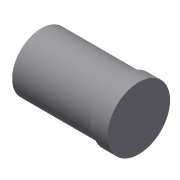
# Autodesk Inventor part: 00_Berrybase_CCTVLens_100mm
Saved by Autodesk Inventor 2022 (Build 260153000, 153)
## iProperties
Created: 2022-08-01
Part Number: 00_Berrybase_CCTVLens_100mm
Material: Generisch
Document SubType Name: Modeling
Designer: diederichbenedict
Density: 1 g/cm^3
Appearance: Vorgabe
Author: diederichbenedict
Autodesk Inventor part; units mm, degrees
ref_plane "YZ Plane" through (0, 0, 0) normal (1, 0, 0) x (0, 1, 0)
sketch "Skizze1" plane through (0, 0, 0) normal (0, 1, 0) x (-1, 0, 0)
  line L0 (0, 0) -> (0, -21)
  line L1 (0, -21) -> (9.5, -21)
  line L2 (9.5, -21) -> (13.5, -19.5)
  line L3 (13.5, -19.5) -> (65.5, -19.5)
  line L4 (65.5, -19.5) -> (65.5, -13.7368)
  line L5 (65.5, -13.7368) -> (65.5, -13.7368)
  line L6 (65.5, -13.7368) -> (65.5, 0)
  line L7 (65.5, 0) -> (0, 0)
  dimension "d0" = 21
  dimension "d1" = 9.5
  dimension "d2" = 65.5
  dimension "d3" = 13.5
  dimension "d4" = 19.5
  dimension "d5" = 0
  constraints: 16 end point, 5 perpendicular, 1 parallel, 1 vertical
  measures "d0" distance of L0.start L0.end
  measures "d1" distance of L0.end L1.end
  measures "d2" distance between parallel lines of L0 L6
  measures "d3" horizontal distance of L2.end L0.end
  measures "d4" distance between parallel lines of L7 L3
  measures "d5" distance between parallel lines of L6 L4
revolve "Umdrehung1" add sketch "Skizze1" angle 360 about axis through (-65.5, 0, 0) along (1, 0, 0)
ref_plane "Arbeitsebene1" through (0, 0, 0) normal (0, 1, 0) x (-1, 0, 0)
ref_plane "Arbeitsebene2" through (0, 0, 0) normal (0, 0, 1) x (1, 0, 0)
